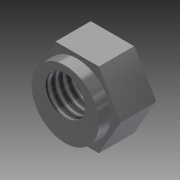
# Autodesk Inventor part: B18033
Saved by Autodesk Inventor 2014 (Build 180170000, 170)
## iProperties
Created: 2013-03-08
Part Number: B18033
Material: Stainless Steel
Document SubType Name: Modeling
Designer: Edward
Density: 1 g/cm^3
Stock Number: B18033
Vendor: custom
Description: Eccentric Nut
Appearance: Semi-Polished
d2: 0.313 in
d3: 0.157 in
d4: 0.00 deg
d5: 0.280 in
d6: 0.050 in
d7: 0.00 deg
d10: 0.165 in
d11: 0.031 in
d21: 0.010 in
Author: Edward
Autodesk Inventor part; units mm, degrees
ref_plane "YZ Plane" through (0, 0, 0) normal (1, 0, 0) x (0, 1, 0)
ref_plane "XZ Plane" through (0, 0, 0) normal (0, 1, 0) x (-1, 0, 0)
ref_plane "XY Plane" through (0, 0, 0) normal (0, 0, 1) x (1, 0, 0)
sketch "Sketch1" plane through (0, 0, 0) normal (0, 0, 1) x (1, 0, 0)
  line L0 (-4.5901, 0) -> (-2.295, 3.9751)
  line L1 (-2.295, 3.9751) -> (2.295, 3.9751)
  line L2 (2.295, 3.9751) -> (4.5901, 0)
  line L3 (4.5901, 0) -> (2.295, -3.9751)
  line L4 (2.295, -3.9751) -> (-2.295, -3.9751)
  line L5 (-2.295, -3.9751) -> (-4.5901, 0)
  point P0 (0, 0)
  dimension "d2" = 7.9502
  constraints: 12 end point, 13 other
  measures "d2" distance between parallel lines of L1 L4
extrude "Extrusion1" add sketch "Sketch1" along normal blind 3.9878
sketch "Sketch2" plane through (0, 0, 3.9878) normal (0, 0, 1) x (1, 0, 0)
  circle A0 centre (0, 0) radius 3.556
  dimension "d5" = 7.112
  constraints: 1 centre point, 1 coincident
  measures "d5" diameter of A0
extrude "Extrusion2" add sketch "Sketch2" along normal blind 1.27
sketch "Sketch3" plane through (0, 0, 5.2578) normal (0, 0, 1) x (1, 0, 0)
  circle A0 centre (0, 0) radius 3.556 projected
  circle A1 centre (0, 0.7874) radius 2.1
  dimension "d10" = 4.2
  dimension "d11" = 0.7874
  constraints: 1 centre point
  measures "d10" diameter of A1
  measures "d11" distance of A0.centre A1.centre
hole "Hole1" at (0, 0.7874, 5.2578) direction (0, 0, -1) diameter 4.1402 end through all
chamfer "Chamfer1" distance 0.254 angle 45 6 edges at (3.4425, -1.9875, 0) (3.4425, 1.9876, 0) (0, 3.9751, 0) (-3.4425, 1.9875, 0) (-3.4425, -1.9876, 0) (0, -3.9751, 0)
body "Solid1"
